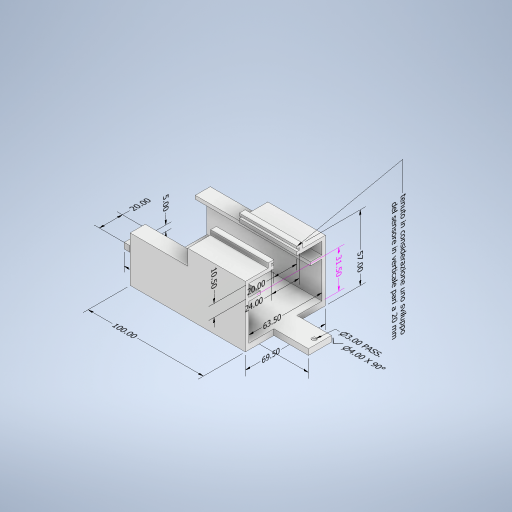
# Autodesk Inventor part: 1
Saved by Autodesk Inventor 2024 (Build 280153000, 153)
## iProperties
Created: 2024-02-08
Part Number: 1
Material: Plastica ABS
Document SubType Name: Modeling
Designer: Pignat Michele
Density: 1.06 g/cm^3
Appearance: Liscia - Bianco
Author: Pignat Michele
Title: SUPPORTO COMPONENTI
Subject: SUPPORTO COMPONENTI
Comments: compontente per ragruppare la componentistica hardware all'interno della box centralina
## iProperties of the stored document pignat_2_Stampa 3D.ipt
Created: 2024-02-09
Part Number: pignat_2_Stampa 3D
Material: Generico
Document SubType Name: Modeling
Designer: user
Density: 1 g/cm^3
Appearance: Default
Author: user
Autodesk Inventor part; units mm, degrees
ref_plane "YZ Plane" through (0, 0, 0) normal (1, 0, 0) x (0, 1, 0)
ref_plane "Piano di lavoro9" through (123.3139, -0.0528, 92.5382) normal (1, 0, 0) x (0, 0, -1)
sketch "Schizzo5" plane through (123.3139, -0.0528, 92.5382) normal (1, 0, 0) x (0, 0, -1)
  line L0 (71.3231, 66.1847) -> (134.8231, 66.1847)
  line L1 (134.8231, 66.1847) -> (134.8231, 34.6847)
  line L2 (134.8231, 34.6847) -> (71.3231, 34.6847)
  line L3 (71.3231, 34.6847) -> (71.3231, 66.1847)
  line L4 (71.3231, 34.6847) -> (81.3231, 34.6847)
  line L5 (81.3231, 34.6847) -> (81.3231, 29.6847)
  line L6 (81.3231, 29.6847) -> (71.3231, 29.6847)
  line L7 (134.8231, 34.6847) -> (124.8231, 34.6847)
  line L8 (124.8231, 34.6847) -> (124.8231, 29.6847)
  line L9 (124.8231, 29.6847) -> (134.8231, 29.6847)
  line L10 (71.3231, 66.1847) -> (81.3231, 66.1847)
  line L11 (81.3231, 66.1847) -> (81.3231, 69.1847)
  line L12 (81.3231, 69.1847) -> (71.3231, 69.1847)
  line L13 (134.8231, 66.1847) -> (124.8231, 66.1847)
  line L14 (124.8231, 66.1847) -> (124.8231, 69.1847)
  line L15 (124.8231, 69.1847) -> (134.8231, 69.1847)
  line L16 (71.3231, 69.1847) -> (68.3231, 69.1847)
  line L17 (68.3231, 69.1847) -> (68.3231, 29.6847)
  line L18 (68.3231, 29.6847) -> (71.3231, 29.6847)
  line L19 (71.3231, 34.6847) -> (71.3231, 66.1847)
  line L20 (134.8231, 69.1847) -> (137.8231, 69.1847)
  line L21 (137.8231, 69.1847) -> (137.8231, 29.6847)
  line L22 (137.8231, 29.6847) -> (134.8231, 29.6847)
  point P0 (92.5382, 0.0528)
  dimension "d18" = 63.5
  dimension "d19" = 31.5
  dimension "d20" = 10
  dimension "d21" = 5
  dimension "d22" = 10
  dimension "d23" = 5
  dimension "d24" = 10
  dimension "d25" = 3
  dimension "d26" = 10
  dimension "d27" = 3
  dimension "d28" = 3
  dimension "d29" = 3
  constraints: 46 end point, 9 parallel, 7 horizontal, 7 perpendicular
  measures "d18" distance of L2.end L1.end
  measures "d19" distance of L1.end L0.end
  measures "d20" distance of L5.end L6.end
  measures "d21" distance of L4.end L5.end
  measures "d22" distance of L9.end L8.end
  measures "d23" distance of L8.end L7.end
  measures "d24" distance of L12.end L11.end
  measures "d25" distance of L11.end L10.end
  measures "d26" distance of L14.end L15.end
  measures "d27" distance of L13.end L14.end
  measures "d28" distance of L18.end L17.end
  measures "d29" distance of L21.end L22.end
extrude "Estrusione3" add sketch "Schizzo5" against normal blind 100 contours L3 L2 L5 L6 L18 L17 L16 L12 L11 L0 | L14 L15 L20 L21 L22 L9 L8 L2 L1 L0
ref_plane "Piano di lavoro11" through (123.3139, -0.0528, 92.5382) normal (1, 0, 0) x (0, 0, -1)
sketch "Schizzo6" plane through (123.3139, -0.0528, 92.5382) normal (1, 0, 0) x (0, 0, -1)
  line L0 (71.3231, 66.1847) -> (81.3231, 66.1847) projected
  line L1 (81.3231, 34.6847) -> (71.3231, 34.6847) projected
  line L2 (81.3231, 29.6847) -> (81.3231, 34.6847) projected
  line L3 (134.8231, 66.1847) -> (134.8231, 34.6847) projected
  line L4 (71.3231, 34.6847) -> (71.3231, 66.1847) projected
  line L5 (68.3231, 99.6847) -> (137.155, 99.6847)
  line L6 (124.8231, 69.1847) -> (137.8231, 69.1847) projected
  line L7 (137.8231, 69.1847) -> (134.8231, 69.1847)
  line L8 (134.8231, 69.1847) -> (134.8231, 79.6847)
  line L9 (137.8231, 79.6847) -> (137.8231, 69.1847)
  line L10 (71.3231, 69.1847) -> (71.3231, 79.6847)
  line L11 (68.3231, 79.6847) -> (68.3231, 69.1847)
  line L12 (115.0731, 79.6847) -> (134.8231, 79.6847)
  line L13 (137.8231, 79.6847) -> (137.8231, 82.6847)
  line L14 (137.8231, 82.6847) -> (118.0731, 82.6847)
  line L15 (91.0731, 79.6847) -> (71.3231, 79.6847)
  line L16 (68.3231, 79.6847) -> (68.3231, 82.6847)
  line L17 (68.3231, 82.6847) -> (88.0731, 82.6847)
  line L18 (91.0731, 82.6847) -> (93.0731, 82.6847)
  line L19 (93.0731, 82.6847) -> (93.0731, 79.6847)
  line L20 (93.0731, 79.6847) -> (91.0731, 79.6847)
  line L21 (115.0731, 82.6847) -> (113.0731, 82.6847)
  line L22 (113.0731, 82.6847) -> (113.0731, 79.6847)
  line L23 (113.0731, 79.6847) -> (115.0731, 79.6847)
  line L24 (91.0731, 82.6847) -> (91.0731, 84.6847)
  line L25 (88.0731, 82.6847) -> (88.0731, 85.6847)
  line L26 (93.0731, 85.6847) -> (93.0731, 84.6847)
  line L27 (93.0731, 84.6847) -> (91.0731, 84.6847)
  line L28 (113.0731, 84.6847) -> (115.0731, 84.6847)
  line L29 (93.0731, 85.6847) -> (93.0731, 86.6847)
  line L30 (88.0731, 85.6847) -> (88.0731, 86.6847)
  line L31 (88.0731, 86.6847) -> (93.0731, 86.6847)
  line L32 (113.0731, 84.6847) -> (113.0731, 86.6847)
  line L33 (113.0731, 86.6847) -> (118.0731, 86.6847)
  line L34 (118.0731, 86.6847) -> (118.0731, 82.6847)
  line L35 (115.0731, 84.6847) -> (115.0731, 82.6847)
  line L36 (68.3231, 69.1847) -> (81.3231, 69.1847) projected
  line L37 (71.3231, 69.1847) -> (68.3231, 69.1847)
  point P0 (92.5382, 0.0528)
  point P1 (68.3231, 29.6847)
  dimension "d32" = 70
  dimension "d33" = 31.5
  dimension "d35" = 63.5
  dimension "d37" = 3
  dimension "d38" = 10.5
  dimension "d39" = 3
  dimension "d40" = 10.5
  dimension "d43" = 3
  dimension "d44" = 3
  dimension "d45" = 2
  dimension "d46" = 2
  dimension "d47" = 2
  dimension "d50" = 2
  dimension "d54" = 2
  dimension "d55" = 4
  dimension "d56" = 5
  dimension "d57" = 2
  dimension "d58" = 2
  dimension "d59" = 5
  constraints: 62 end point, 8 horizontal, 7 perpendicular, 6 parallel, 5 vertical, 1 point on line
  measures "d32" distance of point (68.323, 29.685) L5.start
  measures "d33" distance between parallel lines of L0 L1
  measures "d35" distance between parallel lines of L3 L4
  measures "d37" distance of L8.end L9.start
  measures "d38" distance of L8.end L7.end
  measures "d39" distance of L10.end L11.start
  measures "d40" distance of L10.end L10.start
  measures "d43" distance of L13.end L13.start
  measures "d44" distance of L16.start L16.end
  measures "d45" distance of L19.end L20.end
  measures "d46" distance of L23.end L22.end
  measures "d47" distance of L18.end L26.end
  measures "d50" distance of L21.end L28.start
  measures "d54" distance of L29.end L26.end
  measures "d55" distance between parallel lines of L31 L17
  measures "d56" distance between parallel lines of L29 L30
  measures "d57" distance between parallel lines of L24 L19
  measures "d58" distance of L28.start L32.end
  measures "d59" distance of L32.end L33.end
extrude "Estrusione4" add sketch "Schizzo6" against normal blind 50
sketch "Schizzo7" plane through (123.3139, 29.6319, -32.2849) normal (0, 0, 1) x (1, 0, 0)
  line L0 (0, 5) -> (0, 0) projected
  line L1 (0, 5) -> (-100, 5) projected
  line L2 (-100, 0) -> (-100, 5) projected
  line L3 (0, 0) -> (-100, 0) projected
  point P0 (-123.3139, -29.6319)
extrude "Estrusione5" add sketch "Schizzo7" along normal blind 47.25
sketch "Schizzo8" plane through (123.3139, -0.0528, 92.5382) normal (1, 0, 0) x (0, 0, -1)
  line L0 (71.3231, 66.1847) -> (71.3231, 34.6847) projected
  line L1 (71.3231, 34.6847) -> (65.0934, 34.6847)
  line L2 (134.8231, 34.6847) -> (141.848, 34.6847)
  line L3 (137.8231, 29.6847) -> (137.8231, 82.6847) projected
  line L4 (68.3231, 29.6847) -> (68.3231, 69.1847) projected
  line L5 (137.8231, 34.6847) -> (68.3231, 34.6847)
  line L6 (68.3231, 34.6847) -> (68.3231, 29.6797)
  line L7 (137.8231, 29.6797) -> (137.8231, 34.6847)
  line L8 (68.3231, 29.6847) -> (137.86, 29.6847)
  line L9 (93.0823, 34.6854) -> (113.0823, 34.6854)
  line L10 (113.0823, 34.6854) -> (113.0823, 29.6854)
  line L11 (113.0823, 29.6854) -> (93.0823, 29.6854)
  line L12 (93.0823, 29.6854) -> (93.0823, 34.6854)
  line L13 (113.0823, 34.6854) -> (93.0823, 34.6854)
  line L14 (93.0823, 34.6854) -> (93.0823, 29.6854)
  line L15 (93.0823, 29.6854) -> (113.0823, 29.6854)
  line L16 (113.0823, 29.6854) -> (113.0823, 34.6854)
  point P0 (92.5382, 0.0528)
  point P1 (103.0823, 32.1854)
  point P2 (103.0823, 32.1854)
  point P3 (113.0823, 34.6847)
  point P4 (93.0823, 34.6847)
  dimension "d82" = 20
  dimension "d83" = 5
  constraints: 28 end point, 5 horizontal, 5 parallel, 3 perpendicular, 3 point on line
  measures "d82" distance of L10.end L11.end
  measures "d83" distance of L9.end L10.end
extrude "Estrusione6" add sketch "Schizzo8" along normal blind 25 contours L5 L10 L8 L12
sketch "Schizzo9" plane through (23.3139, -0.0528, 92.5382) normal (-1, 0, 0) x (0, 0, 1)
  line L0 (-71.3231, 66.1847) -> (-71.3231, 34.6847) projected
  line L1 (-71.3231, 34.6847) -> (-67.9708, 34.6847)
  line L2 (-68.3231, 82.6847) -> (-68.3231, 29.6847) projected
  line L3 (-68.3231, 29.6847) -> (-137.8231, 29.6847) projected
  line L4 (-68.3231, 34.6847) -> (-137.8231, 34.6847)
  line L5 (-137.8231, 34.6847) -> (-137.8231, 29.6847)
  line L6 (-137.8231, 29.6847) -> (-68.3231, 29.6847)
  line L7 (-68.3231, 29.6847) -> (-68.3231, 34.6847)
  line L8 (-113.0731, 34.6847) -> (-93.0731, 34.6847)
  line L9 (-93.0731, 34.6847) -> (-93.0731, 29.6847)
  line L10 (-93.0731, 29.6847) -> (-113.0731, 29.6847)
  line L11 (-113.0731, 29.6847) -> (-113.0731, 34.6847)
  point P0 (-92.5382, 0.0528)
  point P1 (-103.0731, 32.1847)
  point P2 (-103.0731, 32.1847)
  dimension "d86" = 20
  dimension "d87" = 5
  constraints: 18 end point, 4 parallel, 3 horizontal, 2 perpendicular, 2 point on line
  measures "d86" distance of L9.end L10.end
  measures "d87" distance of L8.end L9.end
extrude "Estrusione7" add sketch "Schizzo9" along normal blind 25 contours L9 L3 L11 L4
sketch "Schizzo10" plane through (23.3139, 34.6319, 21.2151) normal (0, 1, 0) x (1, 0, 0)
  line L0 (-25, 21.75) -> (-25, 41.75) projected
  line L1 (-25, 31.75) -> (-20, 31.75)
  circle A0 centre (-20, 31.75) radius 0.5
  line L2 (125, 41.7592) -> (125, 21.7592) projected
  line L3 (125, 31.7592) -> (120, 31.7592)
  circle A1 centre (120, 31.7592) radius 0.5
  point P0 (-23.3139, 21.2151)
  dimension "d90" = 5
  dimension "d91" = 1
  dimension "d92" = 5
  dimension "d93" = 1
  constraints: 4 end point, 2 centre point, 2 coincident, 2 horizontal, 2 midpoint
  measures "d90" distance of L1.start L1.end
  measures "d91" diameter of A0
  measures "d92" distance of L3.start L3.end
  measures "d93" diameter of A1
sketch "Schizzo11" plane through (148.3139, -0.0528, 92.5382) normal (1, 0, 0) x (0, 0, -1)
  line L0 (113.0823, 34.6847) -> (93.0823, 34.6847) projected
  line L1 (113.0823, 29.6854) -> (113.0823, 34.6847) projected
  line L2 (93.0823, 34.6847) -> (113.0823, 34.6847)
  line L3 (113.0823, 34.6847) -> (113.0823, 29.6854)
  line L4 (113.0823, 29.6854) -> (93.0823, 29.6854)
  line L5 (93.0823, 29.6854) -> (93.0823, 34.6847)
  point P0 (92.5382, 0.0528)
  constraints: 8 end point, 2 parallel, 1 horizontal, 1 perpendicular
extrude "Estrusione8" add sketch "Schizzo11" along normal blind 5
sketch "Schizzo12" plane through (-1.6861, -0.0528, 92.5382) normal (-1, 0, 0) x (0, 0, 1)
  line L0 (-113.0731, 34.6847) -> (-134.8231, 34.6847) projected
  line L1 (-113.0823, 29.6854) -> (-93.0823, 29.6854) projected
  line L2 (-113.0731, 34.6847) -> (-93.0823, 34.6847)
  line L3 (-93.0823, 34.6847) -> (-93.0823, 29.6854)
  line L4 (-93.0823, 29.6854) -> (-113.0731, 29.6854)
  line L5 (-113.0731, 29.6854) -> (-113.0731, 34.6847)
  point P0 (-92.5382, 0.0528)
  constraints: 8 end point, 2 parallel, 1 horizontal, 1 perpendicular
extrude "Estrusione9" add sketch "Schizzo12" along normal blind 5
hole "Foro3" at (-1.6861, 34.6319, -10.5349) direction (0, -1, 0) diameter 3 end through all countersink diameter 4 countersink angle 90
sketch "Schizzo13" plane through (23.3139, 34.6319, 21.2151) normal (0, 1, 0) x (1, 0, 0)
  line L0 (130, 41.7592) -> (130, 21.7592) projected
  line L1 (130, 31.7592) -> (125, 31.7592)
  point P0 (-23.3139, 21.2151)
  dimension "d133" = 5
  constraints: 2 end point, 1 horizontal, 1 midpoint
  measures "d133" distance of L1.start L1.end
hole "Foro4" at (148.3139, 34.6319, -10.5442) direction (0, -1, 0) diameter 3 end through all countersink diameter 4 countersink angle 90
